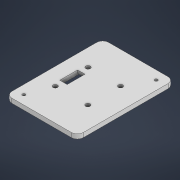
# Autodesk Inventor part: Tampa
Saved by Autodesk Inventor 2022 (Build 260153000, 153)
## iProperties
Created: 2022-07-06
Part Number: Tampa
Material: Generic
Document SubType Name: Modeling
Designer: Gugarauj07
Density: 1 g/cm^3
Appearance: Default
Author: Gugarauj07
Autodesk Inventor part; units mm, degrees
ref_plane "YZ Plane" through (0, 0, 0) normal (1, 0, 0) x (0, 1, 0)
ref_plane "XZ Plane" through (0, 0, 0) normal (0, 1, 0) x (-1, 0, 0)
ref_plane "XY Plane" through (0, 0, 0) normal (0, 0, 1) x (1, 0, 0)
sketch "Sketch1" plane through (0, 0, 0) normal (0, 1, 0) x (-1, 0, 0)
  line L0 (-4, 0) -> (-44, 0)
  line L1 (-48, -4) -> (-48, -61)
  line L2 (-44, -65) -> (-4, -65)
  line L3 (0, -61) -> (0, -4)
  arc A0 (0, -4) -> (-4, 0) centre (-4, -4) ccw
  arc A1 (-4, -65) -> (0, -61) centre (-4, -61) ccw
  arc A2 (-48, -61) -> (-44, -65) centre (-44, -61) ccw
  arc A3 (-44, 0) -> (-48, -4) centre (-44, -4) ccw
  line L4 (-48, -65) -> (-42, -65)
  line L5 (-48, -59) -> (-48, -65)
  line L6 (0, 0) -> (-6, 0)
  line L7 (0, -6) -> (0, 0)
  circle A4 centre (-6, -6) radius 1
  circle A5 centre (-42, -59) radius 1
  line L8 (-14.6534, -26.5) -> (-14.6534, -38.5)
  line L9 (-14.6534, -38.5) -> (-9.6534, -38.5)
  line L10 (-9.6534, -38.5) -> (-9.6534, -26.5)
  line L11 (-9.6534, -26.5) -> (-14.6534, -26.5)
  line L12 (-9.6534, -26.5) -> (-9.6534, -19.5)
  line L13 (-9.6534, -19.5) -> (-35.6534, -19.5)
  line L14 (-35.6534, -19.5) -> (-35.6534, -45.5)
  line L15 (-35.6534, -45.5) -> (-9.6534, -45.5)
  line L16 (-9.6534, -45.5) -> (-9.6534, -19.5)
  point P0 (-48, 0)
  point P1 (0, -65)
  dimension "d0" = 48
  dimension "d1" = 65
  dimension "d3" = 4
  constraints: 34 end point, 8 point on circle, 8 point on line, 8 tangent, 6 centre point, 5 horizontal, 4 parallel, 4 perpendicular, 2 equal radius, 1 vertical
  measures "d0" distance of point (0, -65) L4.start
  measures "d1" distance of L4.start point (-48, 0)
  measures "d3" radius of A1
extrude "Extrusion1" add sketch "Sketch1" along normal blind 3 contours A0 L3 A1 L2 A2 L1 A3 L0
sketch "Sketch3" plane through (0, 3, 0) normal (0, 1, 0) x (1, 0, 0)
  line L0 (9.6534, 19.5) -> (9.6534, 45.5) projected
  line L1 (9.6534, 45.5) -> (9.6534, 38.5)
  line L2 (9.6534, 38.5) -> (14.6534, 38.5)
  line L3 (14.6534, 38.5) -> (14.6534, 26.5)
  line L4 (14.6534, 26.5) -> (9.6534, 26.5)
  line L5 (9.6534, 26.5) -> (9.6534, 38.5)
  line L6 (35.6534, 19.5) -> (9.6534, 19.5) projected
  line L7 (9.6534, 45.5) -> (35.6534, 45.5)
  line L8 (35.6534, 45.5) -> (35.6534, 19.5)
  line L9 (35.6534, 19.5) -> (9.6534, 19.5)
  line L10 (9.6534, 19.5) -> (9.6534, 45.5)
  line L11 (9.6534, 19.5) -> (11.6534, 19.5)
  line L12 (9.6534, 21.5) -> (9.6534, 19.5)
  circle A0 centre (11.6534, 21.5) radius 1.5
  line L13 (35.6534, 45.5) -> (35.6534, 19.5) projected
  line L14 (9.6534, 45.5) -> (35.6534, 45.5) projected
  circle A1 centre (11.6534, 43.5) radius 1.5
  circle A2 centre (33.5528, 21.5) radius 1.5
  circle A3 centre (33.5528, 43.5) radius 1.5
  point P0 (0, 0)
  dimension "d20" = 5
  dimension "d21" = 12
  constraints: 22 end point, 4 centre point, 4 parallel, 3 horizontal, 2 perpendicular, 1 point on line
  measures "d20" distance of L3.end L4.end
  measures "d21" distance of L2.end L3.end
extrude "Extrusion2" add sketch "Sketch3" against normal blind 2 contours L0 L4 L3 L2 L7 L8 L6
body "Solid1"
